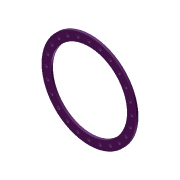
# Autodesk Inventor part: FlyWheelWeight
Saved by Autodesk Inventor 2012 (Build 160160000, 160)
## iProperties
Created: 2012-01-20
Part Number: FlyWheelWeight
Material: Aluminum-6061
Document SubType Name: Modeling
Designer: JesseK
Density: 2.71 g/cm^3
Mass: 132.43 g
Surface Area: 283.123 cm^2
Volume: 48.8672 cm^3
Author: JesseK
Autodesk Inventor part; units mm, degrees
ref_plane "YZ Plane" through (0, 0, 0) normal (1, 0, 0) x (0, 1, 0)
ref_plane "XZ Plane" through (0, 0, 0) normal (0, 1, 0) x (-1, 0, 0)
ref_plane "XY Plane" through (0, 0, 0) normal (0, 0, 1) x (1, 0, 0)
sketch "Sketch1" plane through (0, 0, 0) normal (0, 0, 1) x (1, 0, 0)
  circle A0 centre (0, 0) radius 82.55
  circle A1 centre (0, 0) radius 101.6
  dimension "d0" = 203.2
  dimension "d1" = 19.05
  constraints: 2 centre point, 2 coincident
  measures "d0" diameter of A1
  measures "d1" radial gap between concentric circles of A1 A0
extrude "Extrusion1" add sketch "Sketch1" along normal blind 4.7625
sketch "Sketch2" plane through (0, 0, 4.7625) normal (0, 0, 1) x (1, 0, 0)
  circle A0 centre (0, 0) radius 101.6 projected
  line L0 (0, 0) -> (0, 92.075) construction
  circle A1 centre (0, 0) radius 92.075 construction
  circle A2 centre (0, 92.075) radius 3.175
  dimension "d4" = 9.525
  dimension "d5" = 6.35
  constraints: 2 coincident, 2 end point, 1 centre point, 1 vertical, 1 vertical alignment, 2 other
  measures "d5" diameter of A2
extrude "Extrusion2" cut sketch "Sketch2" against normal through all contours A2
pattern_circular "Circular Pattern1" count 24 over 360 about axis through (0, 0, -10) along (0, 0, 1) of "Extrusion2"
body "Solid1"
